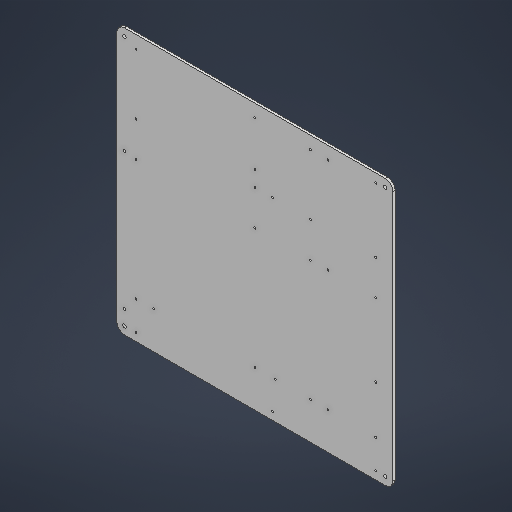
# Autodesk Inventor part: mb_plate_01
Saved by Autodesk Inventor 2026 (Build 300175000, 175)
## iProperties
Created: 2025-01-09
Part Number: mb_plate_01
Material: 一般
Document SubType Name: Modeling
Designer: nyxeon
Density: 1 g/cm^3
Appearance: 既定
Author: nyxeon
Autodesk Inventor part; units mm, degrees
ref_plane "YZ Plane" through (0, 0, 0) normal (1, 0, 0) x (0, 1, 0)
ref_plane "XZ Plane" through (0, 0, 0) normal (0, 1, 0) x (-1, 0, 0)
ref_plane "XY Plane" through (0, 0, 0) normal (0, 0, 1) x (1, 0, 0)
sketch "スケッチ1" plane through (0, 0, 0) normal (0, 0, 1) x (1, 0, 0)
  circle A0 centre (233.68, 2.54) radius 2.25 construction
  circle A1 centre (161.29, 2.54) radius 2.25 construction
  circle A2 centre (29.21, 2.54) radius 2.25 construction
  circle A3 centre (233.68, 160.02) radius 2.25 construction
  circle A4 centre (161.29, 160.02) radius 2.25 construction
  circle A5 centre (6.35, 160.02) radius 2.25 construction
  circle A6 centre (6.35, 284.48) radius 2.25 construction
  circle A7 centre (161.29, 284.48) radius 2.25 construction
  circle A8 centre (233.68, 284.48) radius 2.25 construction
  circle A9 centre (29.21, 2.54) radius 1.25
  circle A10 centre (161.29, 2.54) radius 1.25
  circle A11 centre (233.68, 2.54) radius 1.25
  circle A12 centre (233.68, 160.02) radius 1.25
  circle A13 centre (161.29, 160.02) radius 1.25
  circle A14 centre (6.35, 160.02) radius 1.25
  circle A15 centre (6.35, 284.48) radius 1.25
  circle A16 centre (161.29, 284.48) radius 1.25
  circle A17 centre (233.68, 284.48) radius 1.25
  line L0 (341.25, -45.71) -> (-18.75, -45.71)
  line L1 (-18.75, -45.71) -> (-18.75, 300.99)
  line L2 (-18.75, 300.99) -> (341.25, 300.99)
  line L3 (341.25, 300.99) -> (341.25, -45.71)
  line L4 (331.25, 290.99) -> (-8.75, 290.99) construction
  line L5 (-8.75, 290.99) -> (-8.75, -35.71) construction
  line L6 (-8.75, -35.71) -> (331.25, -35.71) construction
  line L7 (331.25, -35.71) -> (331.25, 290.99) construction
  circle A18 centre (-8.75, 290.99) radius 2.25
  circle A19 centre (331.25, 290.99) radius 2.25
  circle A20 centre (331.25, -35.71) radius 2.25
  circle A21 centre (-8.75, -35.71) radius 2.25
  line L8 (-3.85, -3.82) -> (326.35, -3.82) construction
  line L9 (326.35, -3.82) -> (326.35, 300.98) construction
  line L10 (326.35, 300.98) -> (-3.85, 300.98) construction
  line L11 (-3.85, 300.98) -> (-3.85, -3.82) construction
  circle A22 centre (6.35, 2.54) radius 1.25
  circle A23 centre (6.35, -35.52) radius 1.25
  circle A24 centre (6.35, 205.78) radius 1.25
  circle A25 centre (161.29, 205.78) radius 1.25
  circle A26 centre (161.29, 226.08) radius 1.25
  circle A27 centre (184.15, 205.78) radius 1.25
  circle A28 centre (187.95, 2.54) radius 1.25
  circle A29 centre (233.68, 205.78) radius 1.25
  circle A30 centre (256.55, 284.48) radius 1.25
  circle A31 centre (256.55, 160.02) radius 1.25
  circle A32 centre (256.55, 2.54) radius 1.25
  circle A33 centre (318.75, 289.58) radius 1.25
  circle A34 centre (318.75, 2.54) radius 1.25
  circle A35 centre (318.75, 160.02) radius 1.25
  circle A36 centre (318.75, 205.78) radius 1.25
  circle A37 centre (318.75, 64.78) radius 1.25
  circle A38 centre (184.15, -35.52) radius 1.25
  circle A39 centre (318.75, -35.52) radius 1.25
  line L12 (-5.11, -6.35) -> (-7.56, -6.35) construction
  line L13 (-7.56, 152.33) -> (-5.11, 152.33) construction
  circle A40 centre (-8.75, 162.33) radius 1.6
  circle A41 centre (-8.75, -16.35) radius 1.6
  point P0 (0, 0)
  point P1 (-3.81, 297.18)
  point P2 (0, 300.99)
  point P3 (3.7629, -59.9187)
  point P4 (-8.75, 127.64)
  point P5 (161.25, 300.98)
  point P6 (161.25, 300.99)
  point P7 (-3.85, 148.58)
  dimension "d0" = 2.5
  dimension "d1" = 360
  dimension "d2" = 346.7
  dimension "d5" = 10
  dimension "d6" = 4.5
  dimension "d91" = 304.8
  dimension "d92" = 330.2
  dimension "d93" = 10.2
  dimension "d94" = 16.5
  dimension "d95" = 227.33
  dimension "d97" = 0
  dimension "d98" = 320
  dimension "d99" = 154.94
  dimension "d100" = 124.46
  dimension "d101" = 78.7
  dimension "d102" = 20.3
  dimension "d103" = 177.8
  dimension "d105" = 181.6
  dimension "d106" = 250.2
  dimension "d107" = 312.4
  dimension "d108" = 5.1
  dimension "d109" = 219.7
  dimension "d110" = 10
  dimension "d111" = 10
  dimension "d113" = 3.2
  constraints: 33 centre point, 30 equal radius, 24 end point, 15 vertical alignment, 13 coincident, 13 horizontal alignment, 6 parallel, 4 midpoint, 3 perpendicular, 2 horizontal, 2 point on line, 6 other
  measures "d0" diameter of A9
  measures "d1" distance of L1.end L2.end
  measures "d2" distance of L0.end L1.end
  measures "d5" distance between parallel lines of L2 L4
  measures "d6" diameter of A21
  measures "d91" distance of L10.end L8.start
  measures "d92" distance of L9.end L10.end
  measures "d93" distance from line of A6.centre L11
  measures "d94" distance from line of A6.centre L10
  measures "d95" distance of A8.centre A6.centre
  measures "d97" distance from line of L2 point (0, 300.99)
  measures "d98" distance of A6.centre A23.centre
  measures "d99" distance of A16.centre A6.centre
  measures "d100" distance of A6.centre A5.centre
  measures "d101" distance of A6.centre A24.centre
  measures "d102" distance of A26.centre A25.centre
  measures "d103" distance of A24.centre A27.centre
  measures "d105" distance of A22.centre A28.centre
  measures "d106" distance of A6.centre A30.centre
  measures "d107" horizontal distance of A33.centre A6.centre
  measures "d108" vertical distance of A33.centre A30.centre
  measures "d109" vertical distance of A37.centre A30.centre
  measures "d110" distance from line of L12 A41.centre
  measures "d111" distance from line of A40.centre L13
  measures "d113" diameter of A41
extrude "押し出し1" add sketch "スケッチ1" along normal blind 3
fillet "フィレット3" radius 10 4 edges at (-18.75, -45.71, 1.5) (-18.75, 300.99, 1.5) (341.25, 300.99, 1.5) (341.25, -45.71, 1.5)
